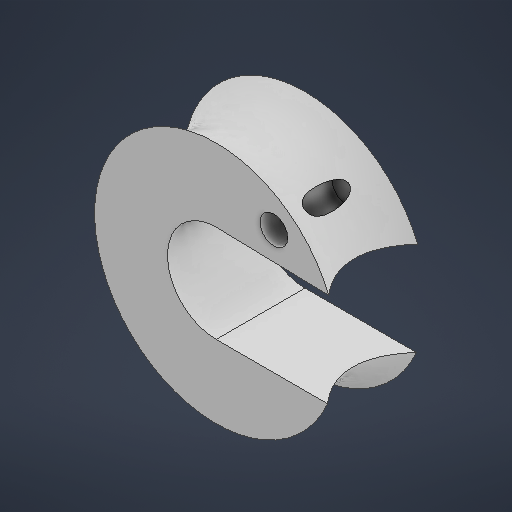
# Autodesk Inventor part: sg90_shaft_support_v2
Saved by Autodesk Inventor 2027 (Build 310192000, 192)
## iProperties
Created: 2026-06-15
Part Number: sg90_shaft_support_v2
Material: Generic
Document SubType Name: Modeling
Designer: alexy
Density: 1 g/cm^3
Appearance: Default
Author: alexy
Autodesk Inventor part; units mm, degrees
ref_plane "YZ Plane" through (0, 0, 0) normal (1, 0, 0) x (0, 1, 0)
ref_plane "XZ Plane" through (0, 0, 0) normal (0, 1, 0) x (-1, 0, 0)
sketch "Sketch1" plane through (0, 0, 0) normal (0, 0, 1) x (1, 0, 0)
  arc A0 (0.0868, 3.4989) -> (0, -3.5) centre (0, 0) ccw
  arc A1 (8.1039, 3.3) -> (8.0195, -3.5) centre (0, 0) ccw
  line L0 (0.0868, 3.4989) -> (8.1039, 3.3)
  line L1 (0, -3.5) -> (8.0195, -3.5)
  dimension "d0" = 7
  dimension "d1" = 17.5
  dimension "d2" = 3.3
  constraints: 4 end point, 4 point on circle, 2 centre point, 2 coincident, 2 tangent, 1 horizontal
  measures "d0" diameter of A0
  measures "d1" diameter of A1
  measures "d2" vertical distance of point (0, 0) L0.end
ref_plane "Work Plane1" through (0, 0, 3.2) normal (0, 0, 1) x (1, 0, 0)
sketch "Sketch2" plane through (0, 0, 3.2) normal (0, 0, 1) x (1, 0, 0)
  arc A0 (6.735, 3.3) -> (6.6332, -3.5) centre (0, 0) ccw
  arc A1 (0.1047, 3.4984) -> (0, -3.5) centre (0, 0) ccw
  line L0 (0.1047, 3.4984) -> (6.735, 3.3)
  line L1 (0, -3.5) -> (6.6332, -3.5)
  dimension "d4" = 15
  dimension "d5" = 7
  dimension "d6" = 3.3
  constraints: 4 end point, 4 point on circle, 2 centre point, 2 coincident, 2 tangent, 1 horizontal
  measures "d4" diameter of A0
  measures "d5" diameter of A1
  measures "d6" vertical distance of point (0, 0) L0.end
ref_plane "Work Plane2" through (0, 0, 6.4) normal (0, 0, 1) x (1, 0, 0)
sketch "Sketch3" plane through (0, 0, 6.4) normal (0, 0, 1) x (1, 0, 0)
  arc A0 (8.1039, 3.3) -> (8.0195, -3.5) centre (0, 0) ccw
  arc A1 (0.0868, 3.4989) -> (0, -3.5) centre (0, 0) ccw
  line L0 (0.0868, 3.4989) -> (8.1039, 3.3)
  line L1 (0, -3.5) -> (8.0195, -3.5)
  dimension "d8" = 17.5
  dimension "d9" = 7
  dimension "d10" = 3.3
  constraints: 5 point on circle, 4 end point, 2 centre point, 2 coincident, 2 tangent, 1 horizontal, 1 point on line
  measures "d8" diameter of A0
  measures "d9" diameter of A1
  measures "d10" vertical distance of point (0, 0) L0.end
loft "Loft1" add profiles "Sketch1", "Sketch2", "Sketch3"
sketch "Sketch4" plane through (0, -3.5, 6.4) normal (0, 0, 1) x (1, 0, 0)
  circle A0 centre (4.1539, 8.8995) radius 1
  line L0 (8.1039, 6.8) -> (0.0868, 6.9989) projected
  point P0 (0, 3.5)
  point P1 (4.0953, 6.8995)
  dimension "d17" = 2
  dimension "d18" = 2
  dimension "d19" = 3.95
  constraints: 1 centre point, 1 midpoint
  measures "d17" diameter of A0
  measures "d18" vertical distance of point (4.095, 6.899) A0.centre
  measures "d19" horizontal distance of L0.start A0.centre
extrude "Extrusion1" cut sketch "Sketch4" against normal blind 5.2
body "Solid1"
